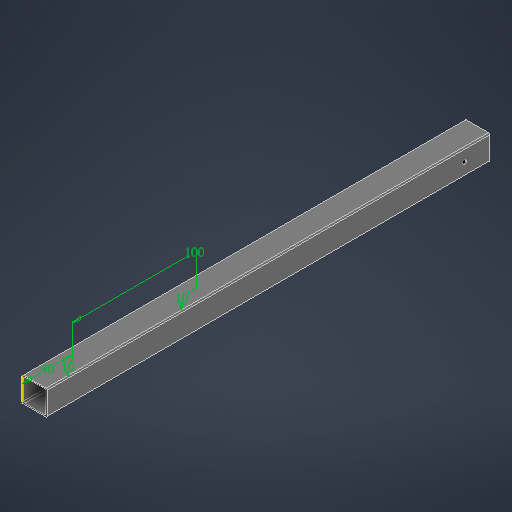
# Autodesk Inventor part: Hlavni_pater
Saved by Autodesk Inventor 2026 (Build 300175050, 175E)
## iProperties
Created: 2026-02-28
Part Number: Hlavni_pater
Material: Všeobecné
Document SubType Name: Modeling
Designer: marti
Density: 1 g/cm^3
Appearance: Šedá
Author: marti
Autodesk Inventor part; units mm, degrees
ref_plane "YZ Plane" through (0, 0, 0) normal (1, 0, 0) x (0, 1, 0)
ref_plane "XZ Plane" through (0, 0, 0) normal (0, 1, 0) x (-1, 0, 0)
ref_plane "XY Plane" through (0, 0, 0) normal (0, 0, 1) x (1, 0, 0)
sketch "Náčrt1" plane through (0, 0, 0) normal (0, 0, 1) x (1, 0, 0)
  line L0 (-10, -10) -> (10, -10)
  line L1 (10, -10) -> (10, 10)
  line L2 (10, 10) -> (-10, 10)
  line L3 (-10, 10) -> (-10, -10)
  line L4 (-10, -10) -> (10, 10) construction
  line L5 (10, -10) -> (-10, 10) construction
  line L6 (-9, -9) -> (9, -9)
  line L7 (9, -9) -> (9, 9)
  line L8 (9, 9) -> (-9, 9)
  line L9 (-9, 9) -> (-9, -9)
  line L10 (-9, -9) -> (9, 9) construction
  line L11 (9, -9) -> (-9, 9) construction
  point P0 (0, 0)
  dimension "d0" = 20
  dimension "d1" = 20
  dimension "d2" = 18
  dimension "d3" = 18
  constraints: 24 end point, 4 midpoint, 4 parallel, 2 horizontal, 2 perpendicular
  measures "d0" distance of L2.end L1.end
  measures "d1" distance of L1.end L0.end
  measures "d2" distance of L8.end L7.end
  measures "d3" distance of L7.end L6.end
extrude "Vysunutí1" add sketch "Náčrt1" along normal mid plane 355
fillet "Zaoblení1" radius 1 8 edges at (-9, -9, 0) (9, -9, 0) (9, 9, 0) (-9, 9, 0) (10, -10, 0) (10, 10, 0) (-10, 10, 0) (-10, -10, 0)
sketch "Náčrt2" plane through (10, -9, 177.5) normal (1, 0, 0) x (0, 0, -1)
  line L0 (355, 18) -> (355, 0) projected
  line L1 (0, -1) -> (355, -1) projected
  point P0 (177.5, 9)
  point P1 (335, 9)
  point P2 (355, 9)
  dimension "d7" = 20
  dimension "d8" = 10
  constraints: 1 midpoint
  measures "d7" distance of point (355, 9) point (335, 9)
  measures "d8" distance from line of L1 point (335, 9)
hole "Díra1" at (10, 0, -157.5) direction (-1, 0, 0) diameter 3 end through all
sketch "Náčrt3" plane through (-10, -9, 177.5) normal (-1, 0, 0) x (0, 0, 1)
  line L0 (0, 18) -> (0, 0) projected
  line L1 (-355, -1) -> (0, -1) projected
  point P0 (-177.5, 9)
  point P1 (-40, 9)
  point P2 (-140, 9)
  dimension "d16" = 40
  dimension "d17" = 10
  dimension "d18" = 100
  dimension "d19" = 10
  measures "d16" distance from line of L0 point (-40, 9)
  measures "d17" distance from line of L1 point (-40, 9)
  measures "d18" distance of point (-140, 9) point (-40, 9)
  measures "d19" distance from line of L1 point (-140, 9)
